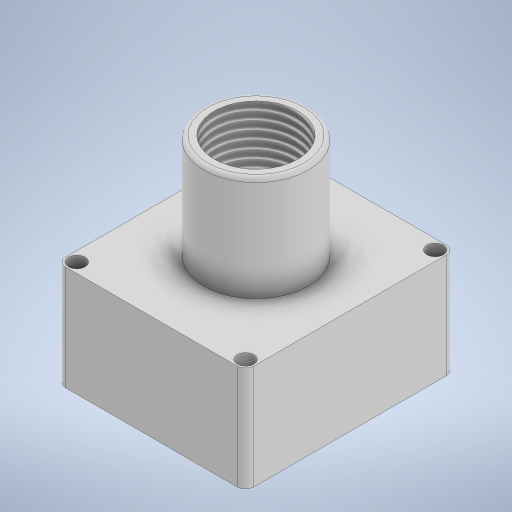
# Autodesk Inventor part: Pieza No.1 Lj
Saved by Autodesk Inventor 2024 (Build 280153000, 153)
## iProperties
Created: 2024-02-18
Part Number: Pieza No.1 Lj
Material: Genérico
Document SubType Name: Modeling
Designer: lejsa
Density: 1 g/cm^3
Appearance: Valor por defecto
Author: lejsa
Autodesk Inventor part; units mm, degrees
ref_plane "YZ Plane" through (0, 0, 0) normal (1, 0, 0) x (0, 1, 0)
ref_plane "XZ Plane" through (0, 0, 0) normal (0, 1, 0) x (-1, 0, 0)
ref_plane "XY Plane" through (0, 0, 0) normal (0, 0, 1) x (1, 0, 0)
sketch "Boceto1" plane through (0, 0, 0) normal (0, 1, 0) x (-1, 0, 0)
  line L0 (-41, 50) -> (41, 50)
  line L1 (45, 46) -> (45, -46)
  line L2 (41, -50) -> (-41, -50)
  line L3 (-45, -46) -> (-45, 46)
  arc A0 (41, -50) -> (45, -46) centre (41, -46) ccw
  arc A1 (45, 46) -> (41, 50) centre (41, 46) ccw
  arc A2 (-41, 50) -> (-45, 46) centre (-41, 46) ccw
  arc A3 (-45, -46) -> (-41, -50) centre (-41, -46) ccw
  line L4 (43.8284, -48.8284) -> (48.8284, -48.8284) construction
  circle A4 centre (40.2929, -45.2929) radius 4
  circle A5 centre (40.2929, 45.2929) radius 4
  circle A6 centre (-40.2929, 45.2929) radius 4
  circle A7 centre (-40.2929, -45.2929) radius 4
  point P0 (0, 0)
  constraints: 10 end point, 9 point on circle, 8 centre point, 8 tangent, 2 horizontal, 2 parallel, 1 perpendicular
extrude "Extrusión1" add sketch "Boceto1" along normal blind 50
sketch "Boceto2" plane through (0, 50, 0) normal (0, 1, 0) x (1, 0, 0)
  circle A0 centre (0, 0) radius 25
  dimension "d19" = 50
  constraints: 1 centre point, 1 coincident
  measures "d19" diameter of A0
extrude "Extrusión2" add sketch "Boceto2" along normal blind 50
sketch "Boceto3" plane through (0, 100, 0) normal (0, 1, 0) x (1, 0, 0)
  circle A0 centre (0, 0) radius 20
  dimension "d22" = 40
  constraints: 1 centre point, 1 coincident
  measures "d22" diameter of A0
extrude "Extrusión3" cut sketch "Boceto3" against normal blind 30
thread "Rosca1" size "M50x4" class "6H" standard "ANSI Metric M Profile" full length
fillet "Empalme1" radius 2 1 edges at (-25, 100, 0)
